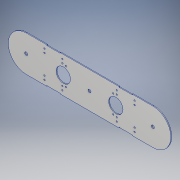
# Autodesk Inventor part: SidePlate
Saved by Autodesk Inventor 2017 (Build 210142000, 142)
## iProperties
Created: 2017-05-20
Part Number: SidePlate
Material: Aluminum 6061
Document SubType Name: Modeling
Designer: steve
Density: 2.7 g/cm^3
Appearance: Aluminum - Flat
Author: steve
Autodesk Inventor part; units mm, degrees
ref_plane "XZ Plane" through (0, 0, 0) normal (0, 1, 0) x (-1, 0, 0)
ref_plane "XY Plane" through (0, 0, 0) normal (0, 0, 1) x (1, 0, 0)
sketch "Sketch1" plane through (0, 0, 0) normal (0, 0, 1) x (1, 0, 0)
  arc A0 (0, 47.625) -> (0, -47.625) centre (0, 0) ccw
  line L0 (-47.625, 0) -> (384.175, 0) construction
  arc A1 (336.55, -47.625) -> (336.55, 47.625) centre (336.55, 0) ccw
  line L1 (0, 47.625) -> (336.55, 47.625)
  line L2 (336.55, -47.625) -> (0, -47.625)
  dimension "d0" = 95.25
  dimension "d1" = 431.8
  dimension "d2" = 95.25
  constraints: 6 end point, 6 point on circle, 3 tangent, 2 centre point, 1 coincident, 1 horizontal, 1 point on line
  measures "d0" diameter of A0
  measures "d1" distance of L0.start L0.end
  measures "d2" diameter of A1
extrude "Extrusion1" add sketch "Sketch1" along normal blind 2.3038
hole "Hole1" at (0, 0, 2.3038) direction (0, 0, -1) diameter 8 end through all
hole "Hole2" at (336.55, 0, 2.3038) direction (0, 0, -1) diameter 8 end through all
sketch "Sketch2" plane through (0, 0, 2.3038) normal (0, 0, 1) x (1, 0, 0)
  circle A0 centre (336.55, 0) radius 4 projected
  circle A1 centre (0, 0) radius 4 projected
  line L0 (336.55, 0) -> (0, 0) construction
  line L1 (168.275, 0) -> (168.275, -1.5875)
  point P0 (0, 0)
  dimension "d23" = 1.5875
  constraints: 4 end point, 1 horizontal, 1 midpoint, 1 vertical
  measures "d23" distance of L1.start L1.end
hole "Hole3" at (168.275, -1.5875, 2.3038) direction (0, 0, -1) diameter 8 end through all
sketch "Sketch4" plane through (0, 0, 2.3038) normal (0, 0, 1) x (1, 0, 0)
  line L0 (336.55, 47.625) -> (0, 47.625) projected
  line L1 (0, -47.625) -> (336.55, -47.625) projected
  line L2 (168.275, 47.625) -> (168.275, -47.625)
  line L3 (168.275, 0) -> (238.125, 0)
  line L4 (168.275, 0) -> (98.425, 0)
  point P0 (0, 0)
  dimension "d41" = 69.85
  dimension "d42" = 69.85
  constraints: 6 end point, 3 midpoint, 2 horizontal
  measures "d41" distance of L3.start L3.end
  measures "d42" distance of L3.start L4.end
hole "Hole5" at (98.425, 0, 2.3038) at (238.125, 0, 2.3038) direction (0, 0, -1) diameter 38.1 end through all
sketch "Sketch5" plane through (0, 0, 0) normal (0, 0, -1) x (-1, 0, 0)
  line L0 (-89.425, 29) -> (-89.425, 26.5) projected
  arc A0 (-89.925, 26) -> (-89.425, 26.5) centre (-89.925, 26.5) ccw projected
  line L1 (-94.925, 26) -> (-89.925, 26) projected
  arc A1 (-94.925, 26) -> (-95.425, 25.5) centre (-94.925, 25.5) ccw projected
  line L2 (-95.425, 19) -> (-95.425, 25.5) projected
  arc A2 (-95.925, 18.5) -> (-95.425, 19) centre (-95.925, 19) ccw projected
  line L3 (-98.425, 18.5) -> (-95.925, 18.5) projected
  arc A3 (-98.425, 18.5) -> (-98.425, -18.5) centre (-98.425, 0) ccw projected
  line L4 (-95.925, -18.5) -> (-98.425, -18.5) projected
  arc A4 (-95.425, -19) -> (-95.925, -18.5) centre (-95.925, -19) ccw projected
  line L5 (-95.425, -25.5) -> (-95.425, -19) projected
  arc A5 (-95.425, -25.5) -> (-94.925, -26) centre (-94.925, -25.5) ccw projected
  line L6 (-89.925, -26) -> (-94.925, -26) projected
  arc A6 (-89.425, -26.5) -> (-89.925, -26) centre (-89.925, -26.5) ccw projected
  line L7 (-89.425, -26.5) -> (-89.425, -29) projected
  arc A7 (-92.425, -32) -> (-89.425, -29) centre (-92.425, -29) ccw projected
  line L8 (-92.425, -32) -> (-118.425, -32) projected
  arc A8 (-121.425, -29) -> (-118.425, -32) centre (-118.425, -29) ccw projected
  line L9 (-121.425, -29) -> (-121.425, 29) projected
  arc A9 (-118.425, 32) -> (-121.425, 29) centre (-118.425, 29) ccw projected
  line L10 (-118.425, 32) -> (-92.425, 32) projected
  arc A10 (-89.425, 29) -> (-92.425, 32) centre (-92.425, 29) ccw projected
  arc A11 (-105.425, 25.85) -> (-105.425, 22.15) centre (-105.425, 24) ccw projected
  arc A12 (-105.425, 22.15) -> (-105.425, 25.85) centre (-105.425, 24) ccw projected
  arc A13 (-105.425, -22.15) -> (-105.425, -25.85) centre (-105.425, -24) ccw projected
  arc A14 (-105.425, -25.85) -> (-105.425, -22.15) centre (-105.425, -24) ccw projected
  line L11 (-247.125, -29) -> (-247.125, -26.5) projected
  arc A15 (-246.625, -26) -> (-247.125, -26.5) centre (-246.625, -26.5) ccw projected
  line L12 (-241.625, -26) -> (-246.625, -26) projected
  arc A16 (-241.625, -26) -> (-241.125, -25.5) centre (-241.625, -25.5) ccw projected
  line L13 (-241.125, -19) -> (-241.125, -25.5) projected
  arc A17 (-240.625, -18.5) -> (-241.125, -19) centre (-240.625, -19) ccw projected
  line L14 (-238.125, -18.5) -> (-240.625, -18.5) projected
  arc A18 (-238.125, -18.5) -> (-238.125, 18.5) centre (-238.125, 0) ccw projected
  line L15 (-240.625, 18.5) -> (-238.125, 18.5) projected
  arc A19 (-241.125, 19) -> (-240.625, 18.5) centre (-240.625, 19) ccw projected
  line L16 (-241.125, 25.5) -> (-241.125, 19) projected
  arc A20 (-241.125, 25.5) -> (-241.625, 26) centre (-241.625, 25.5) ccw projected
  line L17 (-246.625, 26) -> (-241.625, 26) projected
  arc A21 (-247.125, 26.5) -> (-246.625, 26) centre (-246.625, 26.5) ccw projected
  line L18 (-247.125, 26.5) -> (-247.125, 29) projected
  arc A22 (-244.125, 32) -> (-247.125, 29) centre (-244.125, 29) ccw projected
  line L19 (-244.125, 32) -> (-218.125, 32) projected
  arc A23 (-215.125, 29) -> (-218.125, 32) centre (-218.125, 29) ccw projected
  line L20 (-215.125, 29) -> (-215.125, -29) projected
  arc A24 (-218.125, -32) -> (-215.125, -29) centre (-218.125, -29) ccw projected
  line L21 (-218.125, -32) -> (-244.125, -32) projected
  arc A25 (-247.125, -29) -> (-244.125, -32) centre (-244.125, -29) ccw projected
  arc A26 (-231.125, -25.85) -> (-231.125, -22.15) centre (-231.125, -24) ccw projected
  arc A27 (-231.125, -22.15) -> (-231.125, -25.85) centre (-231.125, -24) ccw projected
  arc A28 (-231.125, 22.15) -> (-231.125, 25.85) centre (-231.125, 24) ccw projected
  arc A29 (-231.125, 25.85) -> (-231.125, 22.15) centre (-231.125, 24) ccw projected
  point P0 (0, 0)
extrude "Extrusion2" cut sketch "Sketch5" against normal through all contours A12 A11 | A14 A13 | A27 A26 | A29 A28
ref_plane "Work Plane1" through (168.275, -1.5875, 2.3038) normal (1, 0, 0) x (0, 1, 0)
sketch "Sketch7" plane through (0, 0, 0) normal (0, 0, -1) x (-1, 0, 0)
  point P0 (0, 0)
sketch "Sketch8" plane through (0, 0, 2.3038) normal (0, 0, 1) x (1, 0, 0)
  arc A0 (286.775, -21.025) -> (284.775, -23.025) centre (286.775, -23.025) ccw projected
  line L0 (284.775, -45.625) -> (284.775, -23.025) projected
  line L1 (294.275, -45.625) -> (284.775, -45.625) projected
  line L2 (294.275, -45.625) -> (294.275, -23.025) projected
  arc A1 (294.275, -23.025) -> (292.275, -21.025) centre (292.275, -23.025) ccw projected
  line L3 (292.275, -21.025) -> (286.775, -21.025) projected
  circle A2 centre (288.025, -36.025) radius 1.85 projected
  circle A3 centre (288.025, -26.025) radius 1.85 projected
  arc A4 (243.775, -23.025) -> (241.775, -21.025) centre (241.775, -23.025) ccw projected
  line L4 (241.775, -21.025) -> (236.275, -21.025) projected
  arc A5 (236.275, -21.025) -> (234.275, -23.025) centre (236.275, -23.025) ccw projected
  line L5 (234.275, -45.625) -> (234.275, -23.025) projected
  line L6 (243.775, -45.625) -> (234.275, -45.625) projected
  line L7 (243.775, -45.625) -> (243.775, -23.025) projected
  circle A6 centre (240.525, -36.025) radius 1.85 projected
  circle A7 centre (240.525, -26.025) radius 1.85 projected
  arc A8 (94.775, -21.025) -> (92.775, -23.025) centre (94.775, -23.025) ccw projected
  line L8 (92.775, -45.625) -> (92.775, -23.025) projected
  line L9 (102.275, -45.625) -> (92.775, -45.625) projected
  line L10 (102.275, -45.625) -> (102.275, -23.025) projected
  arc A9 (102.275, -23.025) -> (100.275, -21.025) centre (100.275, -23.025) ccw projected
  line L11 (100.275, -21.025) -> (94.775, -21.025) projected
  circle A10 centre (96.025, -36.025) radius 1.85 projected
  circle A11 centre (96.025, -26.025) radius 1.85 projected
  arc A12 (51.775, -23.025) -> (49.775, -21.025) centre (49.775, -23.025) ccw projected
  line L12 (49.775, -21.025) -> (44.275, -21.025) projected
  arc A13 (44.275, -21.025) -> (42.275, -23.025) centre (44.275, -23.025) ccw projected
  line L13 (42.275, -45.625) -> (42.275, -23.025) projected
  line L14 (51.775, -45.625) -> (42.275, -45.625) projected
  line L15 (51.775, -45.625) -> (51.775, -23.025) projected
  circle A14 centre (48.525, -36.025) radius 1.85 projected
  circle A15 centre (48.525, -26.025) radius 1.85 projected
  point P0 (0, 0)
extrude "Extrusion4" cut sketch "Sketch8" against normal through all contours A2 | A3 | A6 | A7 | A10 | A11 | A14 | A15
sketch "Sketch9" plane through (0, 0, 2.3038) normal (0, 0, 1) x (1, 0, 0)
  line L0 (0, -47.625) -> (336.55, -47.625) projected
  line L1 (54.775, -49.225) -> (54.775, -46.025)
  line L2 (54.775, -46.025) -> (89.775, -46.025)
  line L3 (89.775, -46.025) -> (89.775, -49.225)
  line L4 (54.775, -47.625) -> (89.775, -47.625)
  point P0 (0, 0)
  dimension "d57" = 3.2
  constraints: 8 end point, 2 midpoint, 1 horizontal, 1 perpendicular, 1 vertical, 2 other
  measures "d57" distance of L1.start L1.end
extrude "Extrusion5" cut sketch "Sketch9" against normal through all
mirror "Mirror2" about plane through (168.275, -1.5875, 2.3038) normal (1, 0, 0) of "Extrusion5"
ref_plane "Work Plane2" through (0, 0, 0) normal (0, 1, 0) x (1, 0, 0)
mirror "Mirror3" about plane through (0, 0, 0) normal (0, 1, 0) of "Extrusion4", "Extrusion5", "Mirror2"
body "Solid1"
